# Autodesk Inventor part: bottom
Saved by Autodesk Inventor 2021 (Build 250183000, 183)
## iProperties
Created: 2021-01-15
Part Number: bottom
Material: ABS Plastic
Document SubType Name: Modeling
Designer: User
Density: 1.06 g/cm^3
Appearance: Smooth - Black
Author: User
Autodesk Inventor part; units mm, degrees
ref_plane "YZ Plane" through (0, 0, 0) normal (1, 0, 0) x (0, 1, 0)
ref_plane "XZ Plane" through (0, 0, 0) normal (0, 1, 0) x (-1, 0, 0)
ref_plane "XY Plane" through (0, 0, 0) normal (0, 0, 1) x (1, 0, 0)
sketch "Sketch1" plane through (0, 0, 0) normal (0, 1, 0) x (-1, 0, 0)
  line L0 (-33, 47.5) -> (33, 47.5)
  line L1 (33, 47.5) -> (33, -47.5)
  line L2 (33, -47.5) -> (-33, -47.5)
  line L3 (-33, -47.5) -> (-33, 47.5)
  line L4 (-33, 47.5) -> (33, -47.5) construction
  line L5 (33, 47.5) -> (-33, -47.5) construction
  circle A0 centre (24.5, 39) radius 1.3
  circle A1 centre (24.5, -19) radius 1.3
  circle A2 centre (-24.5, 39) radius 1.3
  circle A3 centre (-24.5, -19) radius 1.3
  line L6 (29, 43.5) -> (-29, 43.5)
  line L7 (-29, 43.5) -> (-29, -43.5)
  line L8 (-29, -43.5) -> (29, -43.5)
  line L9 (29, -43.5) -> (29, 43.5)
  line L10 (29, 43.5) -> (-29, -43.5) construction
  line L11 (-29, 43.5) -> (29, -43.5) construction
  line L12 (18.550301, 43.5) -> (-11.679483, 43.5) construction
  point P0 (0, 0)
  point P1 (-29, 36)
  point P2 (-29, -16)
  dimension "d0" = 66
  dimension "d1" = 95
  dimension "d14" = 2.6
  dimension "d17" = 58
  dimension "d20" = 49
  dimension "d24" = 24.5
  dimension "d25" = 58
  dimension "d26" = 87
  dimension "d27" = 4.5
  dimension "d66" = 4.5
  dimension "d68" = 4.5
  constraints: 26 end point, 4 centre point, 4 horizontal, 4 midpoint, 4 parallel, 2 perpendicular, 2 point on line, 1 vertical, 6 other
  measures "d0" distance of L1.end L2.end
  measures "d1" distance of L0.end L1.end
  measures "d14" diameter of A0
  measures "d17" distance of A0.centre A1.centre
  measures "d20" distance of A0.centre A2.centre
  measures "d24" horizontal distance of point (0, 0) A0.centre
  measures "d25" distance of L8.end L7.end
  measures "d26" distance of L7.end L6.end
  measures "d27" distance from line of L6 A0.centre
  measures "d66" distance from line of L7 A2.centre
  measures "d68" distance from line of A0.centre L12
sketch "Sketch1 outline for base" plane through (0, 0, 0) normal (0, 1, 0) x (-1, 0, 0)
  line L0 (-29, 43.5) -> (-29, -43.5)
  line L1 (29, 43.5) -> (-29, 43.5)
  line L2 (-29, -43.5) -> (29, -43.5)
  line L3 (29, -43.5) -> (29, 43.5)
  circle A0 centre (-24.5, -19) radius 1.3
  circle A1 centre (24.5, -19) radius 1.3
  circle A2 centre (-24.5, 39) radius 1.3
  circle A3 centre (24.5, 39) radius 1.3
extrude "base" add sketch "Sketch1 outline for base" along normal blind 2
sketch "Sketch1 outline for walls" plane through (0, 0, 0) normal (0, 1, 0) x (-1, 0, 0)
  line L0 (-33, 47.5) -> (-33, -47.5)
  line L1 (33, 47.5) -> (-33, 47.5)
  line L2 (-33, -47.5) -> (33, -47.5)
  line L3 (33, -47.5) -> (33, 47.5)
  line L4 (29, -43.5) -> (-29, -43.5)
  line L5 (29, 43.5) -> (29, -43.5)
  line L6 (-29, 43.5) -> (29, 43.5)
  line L7 (-29, -43.5) -> (-29, 43.5)
extrude "walls" add sketch "Sketch1 outline for walls" along normal blind 9.2
fillet "inside" radius 3 3 edges at (-29, 5.6, -43.5) (-29, 5.6, 43.5) (29, 5.6, 43.5)
fillet "outside" radius 7 4 edges at (-33, 4.6, -47.5) (33, 4.6, -47.5) (33, 4.6, 47.5) (-33, 4.6, 47.5)
sketch "cutout_usb_sketch" plane through (0, 0, 0) normal (0, -1, 0) x (1, 0, 0)
  line L0 (26, -47.5) -> (-26, -47.5) projected
  line L1 (25.6, -47.5) -> (25.6, -30.48)
  line L2 (33, 40.5) -> (33, -40.5) projected
  line L3 (25.6, -30.48) -> (10.8, -30.48)
  line L4 (10.8, -30.48) -> (10.8, -47.5)
  line L5 (25.6, -47.5) -> (10.8, -47.5)
  line L6 (25.6, -43.5) -> (10.8, -43.5)
  line L7 (10.8, -43.5) -> (8.575, -43.5)
  line L8 (8.575, -43.5) -> (8.575, -47.5)
  line L9 (8.575, -47.5) -> (10.8, -47.5)
  line L10 (10.8, -47.5) -> (10.8, -43.5)
  line L11 (25.6, -43.5) -> (27.825, -43.5)
  line L12 (27.825, -43.5) -> (27.825, -47.5)
  line L13 (27.825, -47.5) -> (25.6, -47.5)
  line L14 (25.6, -47.5) -> (25.6, -43.5)
  point P0 (0, 0)
  dimension "d76" = 7.4
  dimension "d77" = 14.8
  dimension "d78" = 17.02
  dimension "d102" = 4
  dimension "d103" = 2.225
  dimension "d104" = 2.225
  constraints: 26 end point, 5 point on line, 4 parallel, 4 perpendicular, 3 horizontal, 1 collinear, 1 horizontal alignment, 1 vertical
  measures "d76" distance between parallel lines of L2 L1
  measures "d77" distance of L1.end L3.end
  measures "d78" distance of L1.start L1.end
  measures "d102" distance between parallel lines of L0 L6
  measures "d103" distance of L6.end L7.end
  measures "d104" distance between parallel lines of L1 L12
sketch "cutout_usb_sketch outline for cutout_usb" plane through (0, 0, 0) normal (0, -1, 0) x (1, 0, 0)
  line L0 (25.6, -30.48) -> (10.8, -30.48)
  line L1 (10.8, -30.48) -> (10.8, -43.5)
  line L2 (10.8, -43.5) -> (8.575, -43.5)
  line L3 (8.575, -43.5) -> (8.575, -47.5)
  line L4 (8.575, -47.5) -> (27.825, -47.5)
  line L5 (27.825, -47.5) -> (27.825, -43.5)
  line L6 (27.825, -43.5) -> (25.6, -43.5)
  line L7 (25.6, -43.5) -> (25.6, -30.48)
extrude "cutout_usb" cut sketch "cutout_usb_sketch outline for cutout_usb" against normal through all
sketch "cutout_usb_sketch outline for cutout_usb_cover" plane through (0, 0, 0) normal (0, -1, 0) x (1, 0, 0)
  line L0 (25.6, -30.48) -> (10.8, -30.48)
  line L1 (25.6, -43.5) -> (25.6, -30.48)
  line L2 (10.8, -43.5) -> (25.6, -43.5)
  line L3 (10.8, -30.48) -> (10.8, -43.5)
extrude "cutout_usb_cover" add sketch "cutout_usb_sketch outline for cutout_usb_cover" against normal up to surface (2 mm away)
sketch "cutout_eth_sketch" plane through (0, 0, 0) normal (0, -1, 0) x (1, 0, 0)
  line L0 (8.575, -47.5) -> (-26, -47.5) projected
  line L1 (8.575, -47.5) -> (-8.175, -47.5)
  line L2 (-8.175, -47.5) -> (-8.175, -24.06)
  line L3 (-7.675, -23.56) -> (8.075, -23.56)
  line L4 (8.575, -24.06) -> (8.575, -47.5)
  arc A0 (-7.675, -23.56) -> (-8.175, -24.06) centre (-7.675, -24.06) ccw
  arc A1 (8.575, -24.06) -> (8.075, -23.56) centre (8.075, -24.06) ccw
  point P0 (0, 0)
  point P1 (-8.175, -23.56)
  point P2 (8.575, -23.56)
  dimension "d84" = 16.75
  dimension "d85" = 23.94
  dimension "d147" = 0.5
  constraints: 9 end point, 4 point on circle, 4 point on line, 4 tangent, 2 centre point, 1 equal radius, 1 horizontal, 1 parallel, 1 perpendicular, 1 vertical
  measures "d84" distance of point (-8.175, -23.56) point (8.575, -23.56)
  measures "d85" distance of point (8.575, -23.56) L0.start
  measures "d147" radius of A0
sketch "cutout_eth_sketch outline for cutout_eth" plane through (0, 0, 0) normal (0, -1, 0) x (1, 0, 0)
  arc A0 (8.575, -24.06) -> (8.075, -23.56) centre (8.075, -24.06) ccw
  line L0 (8.575, -47.5) -> (8.575, -24.06)
  line L1 (-8.175, -47.5) -> (8.575, -47.5)
  line L2 (-8.175, -24.06) -> (-8.175, -47.5)
  arc A1 (-7.675, -23.56) -> (-8.175, -24.06) centre (-7.675, -24.06) ccw
  line L3 (8.075, -23.56) -> (-7.675, -23.56)
extrude "cutout_eth" cut sketch "cutout_eth_sketch outline for cutout_eth" against normal through all
fillet "cutout_eth_and_usb_fillet" radius 2 3 edges at (27.825, 4.6, -47.2579) (8.575, 1, -43.5) (-8.175, 4.6, -47.5)
sketch "cutout_stereo_sketch" plane through (0, 0, 0) normal (0, -1, 0) x (1, 0, 0)
  line L0 (-9.52, -35.865) -> (-21.08, -35.865)
  line L1 (-21.08, -35.865) -> (-21.08, -41.135)
  line L2 (-21.08, -41.135) -> (-9.52, -41.135)
  line L3 (-9.52, -41.135) -> (-9.52, -35.865)
  line L4 (-33, -40.5) -> (-33, 40.5) projected
  line L5 (-21.08, -38.5) -> (-9.52, -38.5) construction
  line L6 (8.575, -47.5) -> (-26, -47.5) projected
  point P0 (0, 0)
  point P1 (-8.175, -47.5)
  dimension "d90" = 11.92
  dimension "d91" = 11.56
  dimension "d93" = 5.27
  dimension "d96" = 9
  constraints: 10 end point, 2 midpoint, 2 parallel, 1 horizontal, 1 perpendicular
  measures "d90" distance between parallel lines of L4 L1
  measures "d91" distance of L0.start L0.end
  measures "d93" distance of L0.end L1.end
  measures "d96" distance between parallel lines of L5 L6
sketch "cutout_stereo_sketch outline for cutout_stereo" plane through (0, 0, 0) normal (0, -1, 0) x (1, 0, 0)
  line L0 (-9.52, -35.865) -> (-21.08, -35.865)
  line L1 (-9.52, -41.135) -> (-9.52, -35.865)
  line L2 (-21.08, -41.135) -> (-9.52, -41.135)
  line L3 (-21.08, -35.865) -> (-21.08, -41.135)
extrude "cutout_stereo" cut sketch "cutout_stereo_sketch outline for cutout_stereo" against normal through all
fillet "cutout_stereo_fillet" radius 0.5 4 edges at (-9.52, 1, -35.865) (-21.08, 1, -35.865) (-21.08, 1, -41.135) (-9.52, 1, -41.135)
sketch "cutout_button_rst_sketch" plane through (0, 0, 0) normal (0, -1, 0) x (1, 0, 0)
  circle A0 centre (-23.898, -37.308) radius 1.5
  line L0 (-33, -40.5) -> (-33, 40.5) projected
  line L1 (8.575, -47.5) -> (-26, -47.5) projected
  point P0 (0, 0)
  point P1 (-8.175, -47.5)
  dimension "d97" = 9.102
  dimension "d98" = 10.192
  dimension "d99" = 3
  constraints: 1 centre point
  measures "d97" distance from line of L0 A0.centre
  measures "d98" distance from line of L1 A0.centre
  measures "d99" diameter of A0
sketch "cutout_button_rst_sketch outline for cutout_button_rst" plane through (0, 0, 0) normal (0, -1, 0) x (1, 0, 0)
  circle A0 centre (-23.898, -37.308) radius 1.5
extrude "cutout_button_rst" cut sketch "cutout_button_rst_sketch outline for cutout_button_rst" against normal through all
sketch "cutout_audio_sketch" plane through (-33, 0, -40.5) normal (-1, 0, 0) x (0, 0, 1)
  line L0 (-7, 9.2) -> (-7, 0)
  circle A0 centre (13.366, 5.65) radius 3.6
  line L1 (0, 9.2) -> (81, 9.2)
  line L2 (16.966, 5.65) -> (16.966, 7.2)
  line L3 (9.766, 5.65) -> (9.766, 7.2)
  line L4 (-3, 9.2) -> (81, 9.2)
  line L5 (18.966, 9.2) -> (23.953806, 9.2)
  line L6 (81, 9.2) -> (0, 9.2)
  line L7 (7.766, 9.2) -> (2.95004, 9.2)
  arc A1 (18.966, 9.2) -> (16.966, 7.2) centre (18.966, 7.2) ccw
  arc A2 (9.766, 7.2) -> (7.766, 9.2) centre (7.766, 7.2) ccw
  point P0 (40.5, 0)
  point P1 (16.966, 9.2)
  point P2 (9.766, 9.2)
  point P3 (9.766, 9.2)
  point P4 (12.768087, 9.2)
  point P5 (13.963913, 9.2)
  dimension "d106" = 7.2
  dimension "d111" = 20.366
  dimension "d112" = 3.55
  dimension "d148" = 2
  constraints: 8 end point, 8 point on line, 6 point on circle, 6 tangent, 3 centre point, 1 equal radius, 1 perpendicular, 1 vertical
  measures "d106" diameter of A0
  measures "d111" distance from line of L0 A0.centre
  measures "d112" distance from line of L1 A0.centre
  measures "d148" radius of A1
sketch "cutout_audio_sketch outline for cutout_audio" plane through (-33, 0, -40.5) normal (-1, 0, 0) x (0, 0, 1)
  arc A0 (13.963913, 9.2) -> (12.768087, 9.2) centre (13.366, 5.65) ccw
  line L0 (12.768087, 9.2) -> (7.766, 9.2)
  arc A1 (7.766, 9.2) -> (9.766, 7.2) centre (7.766, 7.2) cw
  line L1 (9.766, 7.2) -> (9.766, 5.65)
  arc A2 (9.766, 5.65) -> (16.966, 5.65) centre (13.366, 5.65) ccw
  line L2 (16.966, 5.65) -> (16.966, 7.2)
  arc A3 (16.966, 7.2) -> (18.966, 9.2) centre (18.966, 7.2) cw
  line L3 (18.966, 9.2) -> (13.963913, 9.2)
extrude "cutout_audio" cut sketch "cutout_audio_sketch outline for cutout_audio" against normal up to surface (4 mm away)
sketch "cutout_usbc_pwr_sketch" plane through (-33, 0, -40.5) normal (-1, 0, 0) x (0, 0, 1)
  line L0 (-3, 9.2) -> (81, 9.2) projected
  line L1 (24.83, 9.2) -> (37.57, 9.2)
  line L2 (37.57, 9.2) -> (37.57, 5.77)
  line L3 (35.57, 3.77) -> (26.83, 3.77)
  line L4 (24.83, 5.77) -> (24.83, 9.2)
  line L5 (-7, 9.2) -> (-7, 0) projected
  arc A0 (35.57, 3.77) -> (37.57, 5.77) centre (35.57, 5.77) ccw
  arc A1 (24.83, 5.77) -> (26.83, 3.77) centre (26.83, 5.77) ccw
  point P0 (40.5, 0)
  point P1 (37.57, 3.77)
  point P2 (24.83, 3.77)
  dimension "d113" = 31.83
  dimension "d114" = 12.74
  dimension "d117" = 5.43
  dimension "d118" = 2
  constraints: 8 end point, 5 point on line, 4 point on circle, 4 tangent, 2 centre point, 2 parallel, 1 equal radius, 1 horizontal, 1 perpendicular
  measures "d113" distance between parallel lines of L5 L4
  measures "d114" distance of point (37.57, 3.77) point (24.83, 3.77)
  measures "d117" distance of L1.end point (37.57, 3.77)
  measures "d118" radius of A0
sketch "cutout_usbc_pwr_sketch outline for cutout_usbc_pwr" plane through (-33, 0, -40.5) normal (-1, 0, 0) x (0, 0, 1)
  line L0 (37.57, 5.77) -> (37.57, 9.2)
  arc A0 (35.57, 3.77) -> (37.57, 5.77) centre (35.57, 5.77) ccw
  line L1 (26.83, 3.77) -> (35.57, 3.77)
  arc A1 (24.83, 5.77) -> (26.83, 3.77) centre (26.83, 5.77) ccw
  line L2 (24.83, 9.2) -> (24.83, 5.77)
  line L3 (37.57, 9.2) -> (24.83, 9.2)
extrude "cutout_usbc_pwr" cut sketch "cutout_usbc_pwr_sketch outline for cutout_usbc_pwr" against normal up to surface (4 mm away)
sketch "cutout_usbc_data_sketch" plane through (-33, 0, -40.5) normal (-1, 0, 0) x (0, 0, 1)
  line L0 (81, 9.2) -> (0, 9.2) projected
  line L1 (39.73, 9.2) -> (52.47, 9.2)
  line L2 (52.47, 9.2) -> (52.47, 5.77)
  line L3 (50.47, 3.77) -> (41.73, 3.77)
  line L4 (39.73, 5.77) -> (39.73, 9.2)
  line L5 (-7, 9.2) -> (-7, 0) projected
  arc A0 (50.47, 3.77) -> (52.47, 5.77) centre (50.47, 5.77) ccw
  arc A1 (39.73, 5.77) -> (41.73, 3.77) centre (41.73, 5.77) ccw
  point P0 (40.5, 0)
  point P1 (52.47, 3.77)
  point P2 (39.73, 3.77)
  dimension "d119" = 46.73
  dimension "d120" = 12.74
  dimension "d121" = 5.43
  dimension "d122" = 2
  constraints: 8 end point, 5 point on line, 4 point on circle, 4 tangent, 2 centre point, 2 parallel, 1 equal radius, 1 horizontal, 1 perpendicular
  measures "d119" distance between parallel lines of L5 L4
  measures "d120" distance of point (52.47, 3.77) point (39.73, 3.77)
  measures "d121" distance between parallel lines of L0 L3
  measures "d122" radius of A0
sketch "cutout_usbc_data_sketch outline for cutout_usbc_data" plane through (-33, 0, -40.5) normal (-1, 0, 0) x (0, 0, 1)
  arc A0 (50.47, 3.77) -> (52.47, 5.77) centre (50.47, 5.77) ccw
  line L0 (41.73, 3.77) -> (50.47, 3.77)
  arc A1 (39.73, 5.77) -> (41.73, 3.77) centre (41.73, 5.77) ccw
  line L1 (39.73, 9.2) -> (39.73, 5.77)
  line L2 (52.47, 9.2) -> (39.73, 9.2)
  line L3 (52.47, 5.77) -> (52.47, 9.2)
extrude "cutout_usbc_data" cut sketch "cutout_usbc_data_sketch outline for cutout_usbc_data" against normal up to surface (4 mm away)
sketch "cutout_hdmi_sketch" plane through (-33, 0, -40.5) normal (-1, 0, 0) x (0, 0, 1)
  line L0 (-3, 9.2) -> (81, 9.2) projected
  line L1 (55.65, 9.2) -> (74.65, 9.2)
  line L2 (74.65, 9.2) -> (74.65, 5.675)
  line L3 (72.65, 3.675) -> (57.65, 3.675)
  line L4 (55.65, 5.675) -> (55.65, 9.2)
  line L5 (88, 0) -> (88, 9.2) projected
  arc A0 (72.65, 3.675) -> (74.65, 5.675) centre (72.65, 5.675) ccw
  arc A1 (55.65, 5.675) -> (57.65, 3.675) centre (57.65, 5.675) ccw
  point P0 (40.5, 0)
  point P1 (74.65, 3.675)
  point P2 (55.65, 3.675)
  dimension "d125" = 13.35
  dimension "d126" = 19
  dimension "d129" = 5.525
  dimension "d130" = 2
  constraints: 8 end point, 5 point on line, 4 point on circle, 4 tangent, 2 centre point, 2 parallel, 1 equal radius, 1 horizontal, 1 perpendicular
  measures "d125" distance between parallel lines of L5 L2
  measures "d126" distance of point (74.65, 3.675) point (55.65, 3.675)
  measures "d129" distance between parallel lines of L0 L3
  measures "d130" radius of A0
sketch "cutout_hdmi_sketch outline for cutout_hdmi" plane through (-33, 0, -40.5) normal (-1, 0, 0) x (0, 0, 1)
  line L0 (74.65, 5.675) -> (74.65, 9.2)
  arc A0 (72.65, 3.675) -> (74.65, 5.675) centre (72.65, 5.675) ccw
  line L1 (57.65, 3.675) -> (72.65, 3.675)
  arc A1 (55.65, 5.675) -> (57.65, 3.675) centre (57.65, 5.675) ccw
  line L2 (55.65, 9.2) -> (55.65, 5.675)
  line L3 (74.65, 9.2) -> (55.65, 9.2)
extrude "cutout_hdmi" cut sketch "cutout_hdmi_sketch outline for cutout_hdmi" against normal up to surface (4 mm away)
sketch "cutout_gpio_sketch" plane through (0, 0, 0) normal (0, -1, 0) x (1, 0, 0)
  line L0 (21.5, 36.4) -> (27.5, 36.4)
  line L1 (28, 35.9) -> (28, -15.9)
  line L2 (27.5, -16.4) -> (21.5, -16.4)
  line L3 (21, -15.9) -> (21, 35.9)
  line L4 (24.5, 36.4) -> (24.5, -16.4) construction
  circle A0 centre (24.5, 39) radius 1.3 projected
  circle A1 centre (24.5, -19) radius 1.3 projected
  arc A2 (21.5, 36.4) -> (21, 35.9) centre (21.5, 35.9) ccw
  arc A3 (28, 35.9) -> (27.5, 36.4) centre (27.5, 35.9) ccw
  arc A4 (21, -15.9) -> (21.5, -16.4) centre (21.5, -15.9) ccw
  arc A5 (27.5, -16.4) -> (28, -15.9) centre (27.5, -15.9) ccw
  point P0 (0, 0)
  point P1 (21, 36.4)
  point P2 (28, -16.4)
  point P3 (28, 36.4)
  point P4 (21, -16.4)
  dimension "d132" = 7
  dimension "d133" = 2.6
  dimension "d134" = 2.6
  dimension "d150" = 0.5
  constraints: 10 end point, 8 point on circle, 8 point on line, 8 tangent, 4 centre point, 3 equal radius, 2 midpoint, 2 parallel, 1 horizontal, 1 perpendicular, 1 vertical alignment
  measures "d132" distance between parallel lines of L3 L1
  measures "d133" distance from line of A0.centre L0
  measures "d134" distance from line of A1.centre L2
  measures "d150" radius of A2
sketch "cutout_gpio_sketch outline for cutout_gpio" plane through (0, 0, 0) normal (0, -1, 0) x (1, 0, 0)
  arc A0 (28, 35.9) -> (27.5, 36.4) centre (27.5, 35.9) ccw
  line L0 (28, -15.9) -> (28, 35.9)
  arc A1 (27.5, -16.4) -> (28, -15.9) centre (27.5, -15.9) ccw
  line L1 (21.5, -16.4) -> (27.5, -16.4)
  arc A2 (21, -15.9) -> (21.5, -16.4) centre (21.5, -15.9) ccw
  line L2 (21, 35.9) -> (21, -15.9)
  arc A3 (21.5, 36.4) -> (21, 35.9) centre (21.5, 35.9) ccw
  line L3 (27.5, 36.4) -> (21.5, 36.4)
extrude "cutout_gpio" cut sketch "cutout_gpio_sketch outline for cutout_gpio" against normal up to surface (2 mm away)
sketch "cutout_heatsink_sketch" plane through (0, 0, 0) normal (0, -1, 0) x (1, 0, 0)
  line L0 (-10.175, -47.5) -> (-26, -47.5) projected
  line L1 (-26, 47.5) -> (26, 47.5) projected
  line L2 (33, 40.5) -> (33, -40.5) projected
  line L3 (-33, -40.5) -> (-33, 40.5) projected
  line L4 (-18.95, 38.5) -> (19, 38.5)
  line L5 (21, 36.5) -> (21, -5.5)
  line L6 (19, -7.5) -> (-18.95, -7.5)
  line L7 (-20.95, -5.5) -> (-20.95, 36.5)
  line L8 (21.5, 36.4) -> (27.5, 36.4) projected
  arc A0 (21, 36.5) -> (19, 38.5) centre (19, 36.5) ccw
  arc A1 (-18.95, 38.5) -> (-20.95, 36.5) centre (-18.95, 36.5) ccw
  arc A2 (-20.95, -5.5) -> (-18.95, -7.5) centre (-18.95, -5.5) ccw
  arc A3 (19, -7.5) -> (21, -5.5) centre (19, -5.5) ccw
  line L9 (21, -15.9) -> (21, 35.9) projected
  point P0 (0, 0)
  dimension "d165" = 12.05
  dimension "d166" = 9
  dimension "d168" = 40
  dimension "d169" = 2
  dimension "d170" = 0
  constraints: 8 end point, 8 point on circle, 8 tangent, 4 centre point, 3 equal radius, 2 parallel, 1 horizontal, 1 perpendicular
  measures "d165" distance between parallel lines of L3 L7
  measures "d166" distance between parallel lines of L1 L4
  measures "d168" distance between parallel lines of L0 L6
  measures "d169" radius of A0
  measures "d170" distance between parallel lines of L9 L5
sketch "cutout_heatsink_sketch outline for cutout_heatsink" plane through (0, 0, 0) normal (0, -1, 0) x (1, 0, 0)
  arc A0 (-20.95, -5.5) -> (-18.95, -7.5) centre (-18.95, -5.5) ccw
  line L0 (-20.95, 36.5) -> (-20.95, -5.5)
  arc A1 (-18.95, 38.5) -> (-20.95, 36.5) centre (-18.95, 36.5) ccw
  line L1 (19, 38.5) -> (-18.95, 38.5)
  arc A2 (21, 36.5) -> (19, 38.5) centre (19, 36.5) ccw
  line L2 (21, -5.5) -> (21, 36.5)
  arc A3 (19, -7.5) -> (21, -5.5) centre (19, -5.5) ccw
  line L3 (-18.95, -7.5) -> (19, -7.5)
extrude "cutout_heatsink" cut sketch "cutout_heatsink_sketch outline for cutout_heatsink" against normal up to surface (2 mm away)
fillet "cutout_heatsink_gpio_fillet" radius 2 2 edges at (21, 1, 35.9) (21, 1, -5.5)
sketch "cutout_microusb_sketch" plane through (33, 0, 40.5) normal (1, 0, 0) x (0, 0, -1)
  line L0 (70.893, 3.45) -> (63.394, 3.45)
  line L1 (61.394, 5.45) -> (61.394, 9.2)
  line L2 (61.394, 9.2) -> (72.893, 9.2)
  line L3 (72.893, 9.2) -> (72.893, 5.45)
  line L4 (-7, 9.2) -> (-7, 0) projected
  line L5 (0, 9.2) -> (81, 9.2) projected
  arc A0 (70.893, 3.45) -> (72.893, 5.45) centre (70.893, 5.45) ccw
  arc A1 (61.394, 5.45) -> (63.394, 3.45) centre (63.394, 5.45) ccw
  point P0 (40.5, 0)
  point P1 (72.893, 3.45)
  point P2 (61.394, 3.45)
  dimension "d151" = 68.394
  dimension "d152" = 11.499
  dimension "d155" = 0
  dimension "d156" = 5.75
  dimension "d157" = 2
  constraints: 8 end point, 4 point on circle, 4 point on line, 4 tangent, 2 centre point, 2 parallel, 1 equal radius, 1 horizontal, 1 perpendicular
  measures "d151" distance between parallel lines of L4 L1
  measures "d152" distance of point (72.893, 3.45) point (61.394, 3.45)
  measures "d155" distance between parallel lines of L5 L2
  measures "d156" distance of L2.end point (72.893, 3.45)
  measures "d157" radius of A0
sketch "cutout_microusb_sketch outline for cutout_microusb" plane through (33, 0, 40.5) normal (1, 0, 0) x (0, 0, -1)
  arc A0 (61.394, 5.45) -> (63.394, 3.45) centre (63.394, 5.45) ccw
  line L0 (61.394, 9.2) -> (61.394, 5.45)
  line L1 (72.893, 9.2) -> (61.394, 9.2)
  line L2 (72.893, 5.45) -> (72.893, 9.2)
  arc A1 (70.893, 3.45) -> (72.893, 5.45) centre (70.893, 5.45) ccw
  line L3 (63.394, 3.45) -> (70.893, 3.45)
extrude "cutout_microusb" cut sketch "cutout_microusb_sketch outline for cutout_microusb" against normal up to surface (4 mm away)
sketch "cutout_fan_power_sketch" plane through (0, 0, 0) normal (0, -1, 0) x (1, 0, 0)
  line L0 (-8.6, -7.5) -> (-0.6, -7.5)
  line L1 (-0.6, -8.5) -> (-0.6, -12.8)
  line L2 (-1.6, -13.8) -> (-7.6, -13.8)
  line L3 (-8.6, -12.8) -> (-8.6, -8.5)
  line L4 (-10.175, -47.5) -> (-26, -47.5)
  line L5 (33, 40.5) -> (33, -40.5)
  line L6 (19, -7.5) -> (-18.95, -7.5)
  arc A0 (-8.6, -12.8) -> (-7.6, -13.8) centre (-7.6, -12.8) ccw
  arc A1 (-1.6, -13.8) -> (-0.6, -12.8) centre (-1.6, -12.8) ccw
  line L7 (-9.6, -7.5) -> (-15.497155, -7.5)
  line L8 (-18.95, -7.5) -> (19, -7.5)
  line L9 (0.4, -7.5) -> (7.409765, -7.5)
  arc A2 (-8.6, -8.5) -> (-9.6, -7.5) centre (-9.6, -8.5) ccw
  arc A3 (0.4, -7.5) -> (-0.6, -8.5) centre (0.4, -8.5) ccw
  point P0 (0, 0)
  point P1 (-0.6, -13.8)
  point P2 (-8.6, -13.8)
  point P3 (-0.6, -7.5)
  dimension "d172" = 33.7
  dimension "d173" = 8
  dimension "d175" = 33.6
  dimension "d176" = 0
  dimension "d177" = 1
  dimension "d180" = 1
  constraints: 12 end point, 10 point on line, 8 point on circle, 8 tangent, 4 centre point, 2 equal radius, 2 parallel, 1 horizontal, 1 perpendicular
  measures "d172" distance between parallel lines of L4 L2
  measures "d173" distance of point (-0.6, -13.8) point (-8.6, -13.8)
  measures "d175" distance between parallel lines of L5 L1
  measures "d176" distance between parallel lines of L6 L0
  measures "d177" radius of A0
  measures "d180" radius of A2
sketch "cutout_fan_power_sketch outline for cutout_fan_power" plane through (0, 0, 0) normal (0, -1, 0) x (1, 0, 0)
  line L0 (-0.6, -12.8) -> (-0.6, -8.5)
  arc A0 (-1.6, -13.8) -> (-0.6, -12.8) centre (-1.6, -12.8) ccw
  line L1 (-7.6, -13.8) -> (-1.6, -13.8)
  arc A1 (-8.6, -12.8) -> (-7.6, -13.8) centre (-7.6, -12.8) ccw
  line L2 (-8.6, -8.5) -> (-8.6, -12.8)
  arc A2 (-9.6, -7.5) -> (-8.6, -8.5) centre (-9.6, -8.5) cw
  line L3 (-8.6, -7.5) -> (-9.6, -7.5)
  line L4 (-0.6, -7.5) -> (-8.6, -7.5)
  line L5 (0.4, -7.5) -> (-0.6, -7.5)
  arc A3 (-0.6, -8.5) -> (0.4, -7.5) centre (0.4, -8.5) cw
extrude "cutout_fan_power" cut sketch "cutout_fan_power_sketch outline for cutout_fan_power" against normal up to surface (2 mm away)
sketch "Sketch16" plane through (-26, 0, -47.5) normal (0, 0, -1) x (-1, 0, 0)
  line L0 (-5.92, 2.7) -> (-17.825, 2.7)
  line L1 (-17.825, 2.7) -> (-17.825, 9.2)
  line L2 (-17.825, 9.2) -> (-4.92, 9.2)
  line L3 (-4.92, 9.2) -> (-4.92, 3.7)
  line L4 (7, 0) -> (7, 9.2) projected
  line L5 (-17.825, 9.2) -> (-17.825, 0) projected
  line L6 (-15.825, 9.2) -> (0, 9.2) projected
  arc A0 (-5.92, 2.7) -> (-4.92, 3.7) centre (-5.92, 3.7) ccw
  point P0 (-26, 0)
  point P1 (-4.92, 2.7)
  dimension "d181" = 11.92
  dimension "d183" = 0
  dimension "d186" = 0
  dimension "d187" = 6.5
  dimension "d188" = 1
  constraints: 8 end point, 3 point on line, 2 parallel, 2 point on circle, 2 tangent, 1 centre point, 1 horizontal, 1 perpendicular
  measures "d181" distance between parallel lines of L4 L3
  measures "d183" distance between parallel lines of L5 L1
  measures "d186" distance between parallel lines of L6 L2
  measures "d187" distance of L2.end point (-4.92, 2.7)
  measures "d188" radius of A0
sketch "Sketch16 outline for Extrusion22" plane through (-26, 0, -47.5) normal (0, 0, -1) x (-1, 0, 0)
  line L0 (-17.825, 2.7) -> (-5.92, 2.7)
  line L1 (-17.825, 9.2) -> (-17.825, 2.7)
  line L2 (-4.92, 9.2) -> (-17.825, 9.2)
  line L3 (-4.92, 3.7) -> (-4.92, 9.2)
  arc A0 (-5.92, 2.7) -> (-4.92, 3.7) centre (-5.92, 3.7) ccw
extrude "Extrusion22" cut sketch "Sketch16 outline for Extrusion22" against normal up to surface (4 mm away)
equation "\"d14\" = hole"
equation "\"d24\" = 0.5 * d20"
equation "\"hole\" = 2.6"
body "Solid2"
